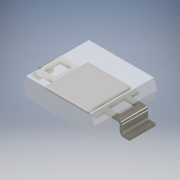
# Autodesk Inventor part: Photodiode_SFH2430
Saved by Autodesk Inventor 2018 (Build 220112000, 112)
## iProperties
Created: 2018-11-29
Part Number: Photodiode_SFH2430
Material: Silver
Document SubType Name: Modeling
Designer: Bradley
Density: 10.49 g/cm^3
Appearance: Silver
Author: Bradley
Autodesk Inventor part; units mm, degrees
ref_plane "YZ Plane" through (0, 0, 0) normal (1, 0, 0) x (0, 1, 0)
ref_plane "XZ Plane" through (0, 0, 0) normal (0, 1, 0) x (-1, 0, 0)
ref_plane "XY Plane" through (0, 0, 0) normal (0, 0, 1) x (1, 0, 0)
sketch "Sketch2" plane through (0, 0, 0) normal (0, 1, 0) x (-1, 0, 0)
  line L0 (3.225, -0.83) -> (2.875, -0.83)
  arc A0 (2.625, -0.58) -> (2.875, -0.83) centre (2.875, -0.58) ccw
  line L1 (2.625, -0.58) -> (2.625, -0.25)
  arc A1 (2.625, -0.25) -> (2.525, -0.15) centre (2.525, -0.25) ccw
  line L2 (2.525, -0.15) -> (-2.525, -0.15)
  arc A2 (-2.525, -0.15) -> (-2.625, -0.25) centre (-2.525, -0.25) ccw
  line L3 (-2.625, -0.25) -> (-2.625, -0.58)
  arc A3 (-2.875, -0.83) -> (-2.625, -0.58) centre (-2.875, -0.58) ccw
  line L4 (-2.875, -0.83) -> (-3.225, -0.83)
  line L5 (-3.225, -0.83) -> (-3.225, -0.68)
  line L6 (-3.225, -0.68) -> (-2.875, -0.68)
  arc A4 (-2.875, -0.68) -> (-2.775, -0.58) centre (-2.875, -0.58) ccw
  line L7 (-2.775, -0.58) -> (-2.775, -0.25)
  arc A5 (-2.525, 0) -> (-2.775, -0.25) centre (-2.525, -0.25) ccw
  line L8 (-2.525, 0) -> (2.525, 0)
  arc A6 (2.775, -0.25) -> (2.525, 0) centre (2.525, -0.25) ccw
  line L9 (2.775, -0.25) -> (2.775, -0.58)
  arc A7 (2.775, -0.58) -> (2.875, -0.68) centre (2.875, -0.58) ccw
  line L10 (2.875, -0.68) -> (3.225, -0.68)
  line L11 (3.225, -0.68) -> (3.225, -0.83)
  point P0 (0, 0)
  point P1 (0, 0)
  point P2 (0, 0)
  dimension "d5" = 0.15
  dimension "d6" = 6.45
  dimension "d7" = 0.83
  dimension "d8" = 0.1
  dimension "d9" = 0.7
  constraints: 24 end point, 16 point on circle, 16 tangent, 10 perpendicular, 8 centre point, 4 concentric, 3 equal radius, 2 coincident, 2 collinear, 1 horizontal, 1 midpoint, 1 parallel
  measures "d5" distance between parallel lines of L0 L10
  measures "d6" distance between parallel lines of L5 L11
  measures "d7" distance between parallel lines of L0 L8
  measures "d8" radius of A1
  measures "d9" distance from line of L8.end L11
extrude "Extrusion2" add sketch "Sketch2" along normal mid plane 2.65
sketch "Sketch3" plane through (-2.525, 1.325, 0) normal (0, 0, 1) x (1, 0, 0)
  line L0 (-0.35, 0) -> (-0.35, -2.65)
  line L1 (-0.7, 0) -> (-0.35, 0)
  line L2 (-0.7, 0) -> (-0.7, -2.65)
  line L3 (-0.35, -2.65) -> (-0.7, -2.65)
  line L4 (-0.25, 0) -> (-0.25, -2.65)
  line L5 (-0.35, 0) -> (-0.25, 0)
  line L6 (-0.35, 0) -> (-0.35, -2.65)
  line L7 (-0.25, -2.65) -> (-0.35, -2.65)
  line L8 (0, 0) -> (0, -2.65)
  line L9 (-0.25, 0) -> (0, 0)
  line L10 (-0.25, 0) -> (-0.25, -2.65)
  line L11 (0, -2.65) -> (-0.25, -2.65)
  line L12 (5.05, 0) -> (5.05, -2.65)
  line L13 (0, 0) -> (5.05, 0)
  line L14 (0, 0) -> (0, -2.65)
  line L15 (5.05, -2.65) -> (0, -2.65)
  line L16 (5.75, 0) -> (5.75, -2.65)
  line L17 (5.4, 0) -> (5.75, 0)
  line L18 (5.4, 0) -> (5.4, -2.65)
  line L19 (5.75, -2.65) -> (5.4, -2.65)
  line L20 (5.4, 0) -> (5.4, -2.65)
  line L21 (5.3, 0) -> (5.4, 0)
  line L22 (5.3, 0) -> (5.3, -2.65)
  line L23 (5.4, -2.65) -> (5.3, -2.65)
  line L24 (5.3, 0) -> (5.3, -2.65)
  line L25 (5.05, 0) -> (5.3, 0)
  line L26 (5.05, 0) -> (5.05, -2.65)
  line L27 (5.3, -2.65) -> (5.05, -2.65)
  line L28 (-0.7, 0) -> (-0.7, -2.65)
  line L29 (-0.7, -0.925) -> (-0.35, -0.925)
  line L30 (-0.35, 0) -> (-0.35, -2.65)
  line L31 (-0.7, -1.725) -> (-0.35, -1.725)
  line L32 (-0.7, -0.925) -> (-0.7, -1.725)
  line L33 (1.075, 0) -> (1.075, -0.525)
  line L34 (1.075, -0.525) -> (0, -0.525)
  line L35 (0, -2.125) -> (1.075, -2.125)
  line L36 (1.075, -2.125) -> (1.075, -2.65)
  line L37 (0, -2.65) -> (5.05, -2.65)
  line L38 (3.725, -2.65) -> (3.725, 0)
  line L39 (0, 0) -> (5.05, 0)
  line L40 (3.925, 0) -> (3.925, -2.65)
  line L41 (4.225, -2.65) -> (4.225, -2.125)
  line L42 (4.225, -2.125) -> (5.75, -2.125)
  line L43 (4.225, 0) -> (4.225, -0.525)
  line L44 (4.225, -0.525) -> (5.75, -0.525)
  line L45 (5.75, -0.525) -> (5.75, -2.125)
  line L46 (5.75, 0) -> (5.75, -2.65)
  line L47 (0, -0.525) -> (0, -2.125)
  line L48 (-0.35, -0.925) -> (0, -0.925)
  line L49 (-0.35, -1.725) -> (0, -1.725)
  point P0 (2.525, -1.325)
  point P1 (5.75, -1.325)
  point P2 (-0.7, -1.325)
extrude "Extrusion4" cut sketch "Sketch3" against normal through all contours L48 L4 L49 L0 | L0 L31 L2 L29 | L48 L8 L49 L4 | L8 L34 L33 L13 L38 L15 L36 L35 | L13 L43 L44 L12 L42 L41 L15 L40 | L44 L22 L42 L12 | L44 L18 L42 L22 | L44 L16 L42 L18 keep common part
sketch "Sketch4" plane through (-1.45, -1.325, 0) normal (0, 0, 1) x (1, 0, 0)
  line L0 (0, 2.125) -> (0, 2.65) projected
  line L1 (-1.075, 2.125) -> (0, 2.125) projected
  line L2 (-1.075, 2.125) -> (-1.075, 1.725) projected
  line L3 (-1.075, 1.725) -> (-1.075, 0.925) projected
  line L4 (-1.075, 0.925) -> (-1.075, 0.525) projected
  line L5 (0, 0.525) -> (-1.075, 0.525) projected
  line L6 (0, 0) -> (0, 0.525) projected
  line L7 (2.65, 0) -> (0, 0) projected
  line L8 (2.65, 2.65) -> (2.65, 0) projected
  line L9 (0, 2.65) -> (2.65, 2.65) projected
  line L10 (0.05, 2.6) -> (2.6, 2.6)
  line L11 (2.6, 2.6) -> (2.6, 0.05)
  line L12 (2.6, 0.05) -> (0.05, 0.05)
  line L13 (0.05, 0.05) -> (0.05, 2.6)
  point P0 (1.45, 1.325)
  point P1 (1.325, 2.6)
  point P2 (1.325, 2.65)
  point P3 (2.6, 1.325)
  point P4 (2.65, 1.325)
  dimension "d22" = 0.05
  dimension "d23" = 0.05
  constraints: 8 end point, 4 midpoint, 2 parallel, 1 horizontal, 1 horizontal alignment, 1 perpendicular, 1 vertical alignment
  measures "d22" distance between parallel lines of L10 L9
  measures "d23" distance between parallel lines of L8 L11
extrude "Extrusion5" cut sketch "Sketch4" against normal blind 0.01 contours L10 L11 L12 L13
sketch "Sketch5" plane through (-1.45, -1.325, 0) normal (0, 0, 1) x (1, 0, 0)
  line L0 (0.05, 0.05) -> (0.05, 2.6) projected
  line L1 (0.05, 2.6) -> (2.6, 2.6) projected
  line L2 (2.6, 2.6) -> (2.6, 0.05) projected
  line L3 (2.6, 0.05) -> (0.05, 0.05) projected
  line L4 (0, 2.125) -> (0, 2.65) projected
  line L5 (-1.075, 2.125) -> (0, 2.125) projected
  line L6 (-1.075, 2.125) -> (-1.075, 1.725) projected
  line L7 (-1.075, 1.725) -> (-1.075, 0.925) projected
  line L8 (-1.075, 0.925) -> (-1.075, 0.525) projected
  line L9 (0, 0.525) -> (-1.075, 0.525) projected
  line L10 (0, 0) -> (0, 0.525) projected
  line L11 (2.65, 0) -> (0, 0) projected
  line L12 (2.65, 2.65) -> (2.65, 0) projected
  line L13 (0, 2.65) -> (2.65, 2.65) projected
  line L14 (3.975, 0.525) -> (3.15, 0.525) projected
  line L15 (3.975, 2.125) -> (3.975, 0.525) projected
  line L16 (3.15, 2.125) -> (3.975, 2.125) projected
  line L17 (3.15, 2.65) -> (3.15, 2.125) projected
  line L18 (2.85, 2.65) -> (3.15, 2.65) projected
  line L19 (2.85, 0) -> (2.85, 2.65) projected
  line L20 (3.15, 0) -> (2.85, 0) projected
  line L21 (3.15, 0.525) -> (3.15, 0) projected
  line L22 (-0.875, 1.825) -> (-0.2, 1.825)
  line L23 (-0.2, 1.825) -> (-0.2, 0.825)
  line L24 (-0.2, 0.825) -> (-0.875, 0.825)
  line L25 (-0.875, 0.825) -> (-0.875, 1.825)
  line L26 (3.05, 1.825) -> (3.775, 1.825)
  line L27 (3.775, 1.825) -> (3.775, 0.825)
  line L28 (3.775, 0.825) -> (3.05, 0.825)
  line L29 (3.05, 0.825) -> (3.05, 1.825)
  point P0 (1.45, 1.325)
  point P1 (-0.5375, 2.125)
  point P2 (-0.5375, 1.825)
  point P3 (-0.2, 1.325)
  dimension "d26" = 0.3
  dimension "d27" = 0.2
  dimension "d28" = 0.2
  dimension "d29" = 0.2
  constraints: 16 end point, 4 parallel, 3 midpoint, 2 horizontal, 2 perpendicular, 1 collinear, 1 horizontal alignment, 1 point on line, 1 vertical alignment
  measures "d26" distance between parallel lines of L5 L22
  measures "d27" distance between parallel lines of L6 L25
  measures "d28" distance between parallel lines of L15 L27
  measures "d29" distance between parallel lines of L19 L29
extrude "Extrusion6" cut sketch "Sketch5" against normal through all contours L22 L23 L24 L25 | L26 L27 L28 L29
sketch "Sketch1" plane through (0, 0, 0) normal (0, 1, 0) x (-1, 0, 0)
  line L0 (2, 0.575) -> (2.2, 0)
  line L1 (2.2, 0) -> (2, -0.575)
  line L2 (2, -0.575) -> (-2, -0.575)
  line L3 (-2, -0.575) -> (-2.2, 0)
  line L4 (-2.2, 0) -> (-2, 0.575)
  line L5 (-2, 0.575) -> (2, 0.575)
  point P0 (0, 0)
  point P1 (0, 0.575)
  point P2 (0, -0.575)
  dimension "d0" = 1.15
  dimension "d1" = 4.4
  dimension "d2" = 4
  constraints: 13 end point, 3 parallel, 2 equal length, 2 midpoint, 2 vertical alignment, 1 horizontal, 1 horizontal alignment
  measures "d0" distance between parallel lines of L2 L5
  measures "d1" distance of L3.end L0.end
  measures "d2" distance of L4.end L0.start
extrude "Extrusion1" add sketch "Sketch1" along normal mid plane 3.85 separate body
equation "\"d23\" = d22"
equation "\"d28\" = d27"
equation "\"d29\" = d28"
body "Solid1"
body "Solid2"
